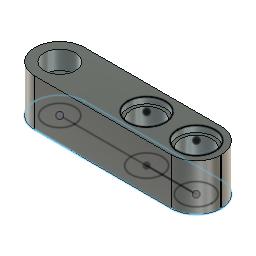
Servo_arm (Autodesk Fusion 360 design; units mm, degrees)
Autodesk Fusion 360 part; units mm, degrees
sketch "Sketch1" plane through (0, 0, 0) normal (0, 0, 1) x (1, 0, 0)
  line L0 (0, 0) -> (22, 0)
  circle A0 centre (22, 0) radius 2.5
  line L1 (22, 0) -> (14, 0)
  circle A1 centre (14, 0) radius 2.5
  circle A2 centre (0, 0) radius 2.4
  line L2 (22.01, -4) -> (-0.01, -4)
  line L3 (-4, -0.01) -> (-4, 0.01)
  line L4 (-0.01, 4) -> (22.01, 4)
  line L5 (26, 0.01) -> (26, -0.01)
  arc A3 (-4, -0.01) -> (-0.01, -4) centre (-0.01, -0.01) ccw
  arc A4 (-0.01, 4) -> (-4, 0.01) centre (-0.01, 0.01) ccw
  arc A5 (26, 0.01) -> (22.01, 4) centre (22.01, 0.01) ccw
  arc A6 (22.01, -4) -> (26, -0.01) centre (22.01, -0.01) ccw
  dimension "d1" = 22
  dimension "d2" = 5
  dimension "d3" = 8
  dimension "d4" = 5
  dimension "d5" = 4.8
  dimension "d6" = 3.99
  dimension "d7" = 3.99
  dimension "d8" = 3.99
  dimension "d9" = 3.99
  constraint coincident L0.start A2.centre
  constraint horizontal L0
  constraint coincident L0.end A0.centre
  constraint parallel L0 L1
  constraint coincident L1.end A1.centre
  constraint horizontal L2
  constraint vertical L3
  constraint horizontal L4
  constraint vertical L5
  constraint tangent L2 A3
  constraint tangent L3 A3
  constraint tangent L3 A4
  constraint tangent L4 A4
  constraint tangent L4 A5
  constraint tangent L5 A5
  constraint tangent L2 A6
  constraint tangent L5 A6
  measures "d1" distance of L0.start L0.end
  measures "d2" diameter of A0
  measures "d3" distance of L0.end L1.end
  measures "d4" diameter of A1
  measures "d5" diameter of A2
  measures "d6" radius of A3
  measures "d7" radius of A4
  measures "d8" radius of A5
  measures "d9" radius of A6
extrude "Extrude1" add sketch "Sketch1" along normal blind 7.5 contours A2 | L2 L3 L4 L5 A3 A4 A5 A6
extrude "Extrude2" cut sketch "Sketch1" along normal blind 2.5 contours A2
sketch "Sketch2" plane through (0, 0, 7.5) normal (0, 0, 1) x (-1, 0, 0)
  circle A0 centre (-22, 0) radius 2.5
  circle A1 centre (-14, 0) radius 2.5
  arc A2 (4, 0.01) -> (0.01, 4) centre (0.01, 0.01) ccw
  line L0 (0.01, 4) -> (-22.01, 4)
  arc A3 (-22.01, 4) -> (-26, 0.01) centre (-22.01, 0.01) ccw
  line L1 (-26, 0.01) -> (-26, -0.01)
  arc A4 (-26, -0.01) -> (-22.01, -4) centre (-22.01, -0.01) ccw
  line L2 (-22.01, -4) -> (0.01, -4)
  arc A5 (0.01, -4) -> (4, -0.01) centre (0.01, -0.01) ccw
  line L3 (4, -0.01) -> (4, 0.01)
  circle A6 centre (0.01, -0.01) radius 1.25
  dimension "d14" = 2.5
  constraint concentric A5 A6
  measures "d14" diameter of A6
extrude "Extrude3" cut sketch "Sketch2" against normal blind 100 contours A6
sketch "Sketch3" plane through (0, 0, 7.5) normal (0, 0, 1) x (-1, 0, 0)
  circle A0 centre (0, 0) radius 2.5
  dimension "d17" = 5
  constraint coincident A0.centre origin
  measures "d17" diameter of A0
extrude "Extrude4" cut sketch "Sketch3" against normal blind 3
sketch "Sketch4" plane through (0, 0, 0) normal (0, 0, 1) x (1, 0, 0)
  circle A0 centre (14, 0) radius 3
  circle A1 centre (22, 0) radius 3
  dimension "d20" = 6
  dimension "d21" = 6
  measures "d20" diameter of A0
  measures "d21" diameter of A1
extrude "Extrude5" cut sketch "Sketch4" along normal blind 1 contours A0
extrude "Extrude6" cut sketch "Sketch4" along normal blind 1 contours A1
sketch "Sketch5" plane through (0, 0, 7.5) normal (0, 0, 1) x (-1, 0, 0)
  circle A0 centre (0, 0) radius 2.5
  circle A1 centre (-22, 0) radius 2.5
  circle A2 centre (-14, 0) radius 2.5
  arc A3 (4, 0.01) -> (0.01, 4) centre (0.01, 0.01) ccw
  line L0 (0.01, 4) -> (-22.01, 4)
  arc A4 (-22.01, 4) -> (-26, 0.01) centre (-22.01, 0.01) ccw
  line L1 (-26, 0.01) -> (-26, -0.01)
  arc A5 (-26, -0.01) -> (-22.01, -4) centre (-22.01, -0.01) ccw
  line L2 (-22.01, -4) -> (0.01, -4)
  arc A6 (0.01, -4) -> (4, -0.01) centre (0.01, -0.01) ccw
  line L3 (4, -0.01) -> (4, 0.01)
  circle A7 centre (-14, 0) radius 3
  circle A8 centre (-22.01, -0.01) radius 3
  dimension "d26" = 6
  dimension "d27" = 6
  constraint concentric A2 A7
  constraint concentric A5 A8
  measures "d26" diameter of A7
  measures "d27" diameter of A8
extrude "Extrude7" cut sketch "Sketch5" against normal blind 1 contours A8
extrude "Extrude8" cut sketch "Sketch5" against normal blind 1 contours A7
